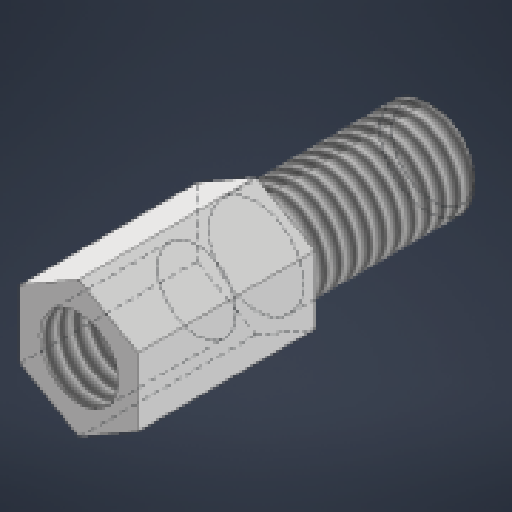
# Autodesk Inventor part: BOLT_STUD_M8_15
Saved by Autodesk Inventor 2023 (Build 270158000, 158)
## iProperties
Created: 2025-09-04
Part Number: BOLT_STUD_M8_15
Material: 일반
Document SubType Name: Modeling
Designer: k
Density: 1 g/cm^3
Appearance: 기본값
Author: k
Autodesk Inventor part; units mm, degrees
ref_plane "YZ Plane" through (0, 0, 0) normal (1, 0, 0) x (0, 1, 0)
ref_plane "XZ Plane" through (0, 0, 0) normal (0, 1, 0) x (-1, 0, 0)
ref_plane "XY Plane" through (0, 0, 0) normal (0, 0, 1) x (1, 0, 0)
sketch "스케치1" plane through (0, 0, 0) normal (0, 0, 1) x (1, 0, 0)
  line L0 (-76.6655, 16.8348) -> (-81.6646, 13.9466)
  line L1 (-81.6646, 13.9466) -> (-86.6655, 16.8319)
  line L2 (-86.6655, 16.8319) -> (-86.6672, 22.6054)
  line L3 (-86.6672, 22.6054) -> (-81.668, 25.4936)
  line L4 (-81.668, 25.4936) -> (-76.6672, 22.6083)
  line L5 (-76.6672, 22.6083) -> (-76.6655, 16.8348)
  point P0 (0, 0)
  point P1 (-81.6663, 19.7201)
  point P2 (-84.1651, 15.3892)
  dimension "d11" = 10
  constraints: 12 end point, 1 midpoint, 13 other
  measures "d11" distance from line of point (-84.165, 15.389) L4
extrude "돌출1" add sketch "스케치1" along normal blind 15
sketch "스케치2" plane through (0, 0, 15) normal (0, 0, 1) x (1, 0, 0)
  line L0 (-76.6655, 16.8348) -> (-76.6672, 22.6083) projected
  line L1 (-81.6646, 13.9466) -> (-76.6655, 16.8348) projected
  point P0 (0, 0)
  point P1 (-81.6663, 19.7201)
  dimension "d14" = 5
  dimension "d15" = 5
  measures "d14" distance from line of L0 point (-81.666, 19.72)
  measures "d15" distance from line of L1 point (-81.666, 19.72)
hole "구멍1" at (-81.6663, 19.7201, 15) direction (0, 0, -1) diameter 6.647 depth 10 thread size "M8x1.25" class "6H" standard "ISO Metric profile"
sketch "스케치3" plane through (0, 0, 0) normal (0, 0, -1) x (-1, 0, 0)
  circle A0 centre (81.6663, 19.7201) radius 4
  line L0 (81.6646, 13.9466) -> (76.6655, 16.8348) projected
  line L1 (76.6672, 22.6083) -> (81.668, 25.4936) projected
  point P0 (0, 0)
  dimension "d23" = 8
  dimension "d24" = 5
  dimension "d25" = 5
  constraints: 1 centre point
  measures "d23" diameter of A0
  measures "d24" distance from line of L0 A0.centre
  measures "d25" distance from line of L1 A0.centre
extrude "돌출2" add sketch "스케치3" along normal blind 15
thread "스레드1" size "M8x1.25" class "6g" standard "ANSI Metric M Profile" full length
chamfer "모따기1" distance 0.5 angle 45 1 edges at (-77.6663, 19.7201, -15)
